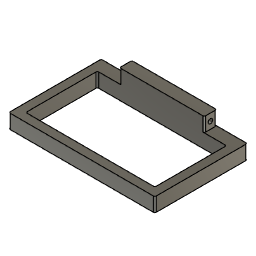
Fire_Base v8 (Autodesk Fusion 360 design; units mm, degrees)
Autodesk Fusion 360 part; units mm, degrees
sketch "Sketch1" plane through (0, 0, 0) normal (0, 0, 1) x (1, 0, 0)
  line L0 (0.5, 0) -> (51.2, 0)
  line L1 (51.7, 0.5) -> (51.7, 32.2)
  line L2 (51.2, 32.7) -> (0.5, 32.7)
  line L3 (0, 32.2) -> (0, 0.5)
  line L4 (51.7, 32.7) -> (0, 0) construction
  line L5 (0, 32.7) -> (51.7, 0) construction
  line L6 (51.7, 16.35) -> (0, 16.35) construction
  line L7 (25.85, 32.7) -> (25.85, 0) construction
  line L8 (51.7, 16.35) -> (48.35, 16.35) construction
  line L9 (0, 16.35) -> (3.35, 16.35) construction
  line L10 (25.85, 0) -> (25.85, 3) construction
  line L11 (25.85, 3) -> (48.2, 3) construction
  line L12 (25.85, 3) -> (0, 3) construction
  line L13 (25.85, 32.7) -> (25.85, 28.35) construction
  line L14 (25.85, 28.35) -> (51.7, 28.35) construction
  line L15 (25.85, 28.35) -> (0, 28.35) construction
  line L16 (3.5, 28.35) -> (48.2, 28.35)
  line L17 (48.7, 27.85) -> (48.7, 3.5)
  line L18 (48.7, 3) -> (3.5, 3)
  line L19 (3, 3.5) -> (3, 27.85)
  arc A0 (0.5, 32.7) -> (0, 32.2) centre (0.5, 32.2) ccw
  arc A1 (3.5, 28.35) -> (3, 27.85) centre (3.5, 27.85) ccw
  arc A2 (3, 3.5) -> (3.5, 3) centre (3.5, 3.5) ccw
  arc A3 (0, 0.5) -> (0.5, 0) centre (0.5, 0.5) ccw
  arc A4 (51.2, 0) -> (51.7, 0.5) centre (51.2, 0.5) ccw
  arc A5 (51.7, 32.2) -> (51.2, 32.7) centre (51.2, 32.2) ccw
  arc A6 (48.7, 27.85) -> (48.2, 28.35) centre (48.2, 27.85) ccw
  arc A7 (48.2, 3) -> (48.7, 3.5) centre (48.2, 3.5) ccw
  point P0 (25.85, 16.35)
  point P1 (48.35, 32.7)
  point P2 (48.35, 0)
  dimension "d1" = 51.7
  dimension "d2" = 32.7
  dimension "d5" = 3
  dimension "d6" = 4.35
  dimension "d7" = 0.5
  dimension "d8" = 0.5
  dimension "d9" = 0.5
  dimension "d10" = 0.5
  dimension "d11" = 0.5
  dimension "d12" = 0.5
  dimension "d13" = 0.5
  dimension "d14" = 0.5
  dimension "d32" = 3
  dimension "d33" = 3
  constraint horizontal L0
  constraint vertical L1
  constraint horizontal L2
  constraint vertical L3
  constraint coincident L4.end origin
  constraint midpoint L4 P0
  constraint perpendicular L1 L8
  constraint perpendicular L3 L9
  constraint perpendicular L0 L10
  constraint perpendicular L1 L11
  constraint coincident L3 L12.end
  constraint perpendicular L3 L12
  constraint perpendicular L11 L13
  constraint coincident L1 L14.end
  constraint perpendicular L1 L14
  constraint coincident L3 L15.end
  constraint perpendicular L3 L15
  constraint horizontal L16
  constraint vertical L17
  constraint horizontal L18
  constraint vertical L19
  constraint coincident L11 L18.start
  constraint coincident L2 L7.start
  constraint coincident L3 L6.end
  constraint coincident L5.start L2
  constraint coincident L5.start L3
  constraint tangent L2 A0
  constraint tangent L3 A0
  constraint tangent L16 A1
  constraint tangent L19 A1
  constraint tangent L18 A2
  constraint tangent L19 A2
  constraint coincident L0 L7.end
  constraint coincident L4.end L0
  constraint coincident L4.end L3
  constraint tangent L0 A3
  constraint tangent L3 A3
  constraint coincident L1 L6.start
  constraint coincident L5.end L0
  constraint coincident L5.end L1
  constraint tangent L0 A4
  constraint tangent L1 A4
  constraint coincident L4.start L2
  constraint coincident L4.start L1
  constraint tangent L2 A5
  constraint tangent L1 A5
  constraint tangent L16 A6
  constraint tangent L17 A6
  constraint coincident L18.start L17
  constraint tangent L17 A7
  constraint tangent L11 A7
  measures "d1" distance of L4.end L5.end
  measures "d2" distance of L4.end L5.start
  measures "d5" distance of L7.end L10.end
  measures "d6" distance of L7.start L13.end
  measures "d7" radius of A0
  measures "d8" radius of A1
  measures "d9" radius of A2
  measures "d10" radius of A3
  measures "d11" radius of A4
  measures "d12" radius of A5
  measures "d13" radius of A6
  measures "d14" radius of A7
  measures "d32" distance of L3 L19
  measures "d33" distance of L1 L17
extrude "Extrude1" add sketch "Sketch1" along normal blind 5
sketch "Sketch2" plane through (0, 0, 5) normal (0, 0, 1) x (-1, 0, 0)
  arc A0 (-3, -3.5) -> (-3.5, -3) centre (-3.5, -3.5) ccw
  line L0 (-3, -3.5) -> (-3, -27.85)
  arc A1 (-3.5, -28.35) -> (-3, -27.85) centre (-3.5, -27.85) ccw
  line L1 (-3.5, -28.35) -> (-48.2, -28.35)
  arc A2 (-48.7, -27.85) -> (-48.2, -28.35) centre (-48.2, -27.85) ccw
  line L2 (-48.7, -27.85) -> (-48.7, -3.5)
  arc A3 (-48.2, -3) -> (-48.7, -3.5) centre (-48.2, -3.5) ccw
  line L3 (-48.2, -3) -> (-3.5, -3)
  arc A4 (-51.7, -32.2) -> (-51.2, -32.7) centre (-51.2, -32.2) ccw
  line L4 (-51.2, -32.7) -> (-0.5, -32.7)
  arc A5 (-0.5, -32.7) -> (0, -32.2) centre (-0.5, -32.2) ccw
  line L5 (0, -32.2) -> (0, -0.5)
  arc A6 (0, -0.5) -> (-0.5, 0) centre (-0.5, -0.5) ccw
  line L6 (-0.5, 0) -> (-51.2, 0)
  arc A7 (-51.2, 0) -> (-51.7, -0.5) centre (-51.2, -0.5) ccw
  line L7 (-51.7, -0.5) -> (-51.7, -32.2)
  line L8 (-51.7, -28.35) -> (0, -28.35) construction
  line L9 (-11.35, -32.7) -> (-40.35, -32.7)
  line L10 (-40.85, -32.2) -> (-40.85, -28.85)
  line L11 (-40.35, -28.35) -> (-11.35, -28.35)
  line L12 (-10.85, -28.85) -> (-10.85, -32.2)
  arc A8 (-11.35, -32.7) -> (-10.85, -32.2) centre (-11.35, -32.2) ccw
  arc A9 (-10.85, -28.85) -> (-11.35, -28.35) centre (-11.35, -28.85) ccw
  arc A10 (-40.85, -32.2) -> (-40.35, -32.7) centre (-40.35, -32.2) ccw
  arc A11 (-40.35, -28.35) -> (-40.85, -28.85) centre (-40.35, -28.85) ccw
  point P0 (-10.85, -32.7)
  point P1 (-40.85, -32.7)
  point P2 (-10.85, -32.7)
  point P3 (-40.85, -32.7)
  point P4 (-10.85, -28.35)
  dimension "d19" = 4.35
  dimension "d20" = 30
  dimension "d21" = 4.35
  dimension "d22" = 0.5
  dimension "d23" = 0.5
  dimension "d24" = 0.5
  dimension "d25" = 0.5
  constraint coincident L7 L8.start
  constraint coincident L5 L8.end
  constraint perpendicular L5 L8
  constraint horizontal L9
  constraint vertical L10
  constraint horizontal L11
  constraint vertical L12
  constraint coincident P2 P0
  constraint coincident P2 L9
  constraint coincident P2 L12
  constraint tangent L9 A8
  constraint tangent L12 A8
  constraint coincident P4 L11
  constraint coincident P4 L12
  constraint tangent L11 A9
  constraint tangent L12 A9
  constraint coincident P3 L9
  constraint coincident P3 L10
  constraint tangent L9 A10
  constraint tangent L10 A10
  constraint tangent L10 A11
  constraint tangent L11 A11
  measures "d19" distance of L4 L8
  measures "d20" distance of P2 P3
  measures "d21" distance of P2 P4
  measures "d22" radius of A8
  measures "d23" radius of A9
  measures "d24" radius of A10
  measures "d25" radius of A11
extrude "Extrude2" add sketch "Sketch2" along normal blind 5 contours L1 L4 L9 L10 L11 L12 A8 A9 A10 A11
sketch "Sketch3" plane through (40.85, 0, 0) normal (1, 0, 0) x (0, 1, 0)
  line L0 (28.85, 5) -> (32.2, 5)
  line L1 (32.2, 5) -> (32.2, 10)
  line L2 (32.2, 10) -> (28.85, 10)
  line L3 (28.85, 10) -> (28.85, 5)
  line L4 (28.85, 10) -> (32.2, 5) construction
  line L5 (32.2, 10) -> (28.85, 5) construction
  line L6 (32.2, 7.5) -> (28.85, 7.5) construction
  circle A0 centre (30.525, 7.5) radius 0.8
  point P0 (30.525, 7.5)
  dimension "d28" = 1.6
  constraint coincident L2.end L3.start
  constraint coincident L0.end L1.start
  constraint coincident L1.end L2.start
  constraint coincident L0.start L3.end
  constraint midpoint L1 L6.start
  constraint midpoint L3 L6.end
  constraint midpoint L6 P0
  constraint coincident P0 A0.centre
  measures "d28" diameter of A0
extrude "Extrude3" cut sketch "Sketch3" against normal blind 40 contours A0
